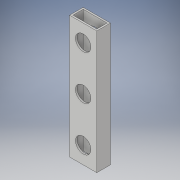
# Autodesk Inventor part: AluminumBar-1111-2020
Saved by Autodesk Inventor 2018 (Build 220112000, 112)
## iProperties
Created: 2020-01-25
Part Number: AluminumBar-1111-2020
Material: Generic
Document SubType Name: Modeling
Designer: Power Hawks CADD
Density: 1 g/cm^3
Appearance: Default
Author: Power Hawks CADD
Autodesk Inventor part; units mm, degrees
ref_plane "YZ Plane" through (0, 0, 0) normal (1, 0, 0) x (0, 1, 0)
ref_plane "XZ Plane" through (0, 0, 0) normal (0, 1, 0) x (-1, 0, 0)
ref_plane "XY Plane" through (0, 0, 0) normal (0, 0, 1) x (1, 0, 0)
sketch "Sketch2" plane through (0, 0, 0) normal (0, 1, 0) x (-1, 0, 0)
  line L0 (0, 0) -> (50.8, 0)
  line L1 (50.8, 0) -> (50.8, -25.4)
  line L2 (50.8, -25.4) -> (0, -25.4)
  line L3 (0, -25.4) -> (0, 0)
  line L4 (47.625, -22.225) -> (47.625, -3.175)
  line L5 (47.625, -3.175) -> (3.175, -3.175)
  line L6 (3.175, -3.175) -> (3.175, -22.225)
  line L7 (3.175, -22.225) -> (47.625, -22.225)
  dimension "d4" = 50.8
  dimension "d5" = 25.4
  dimension "d6" = 3.175
  constraints: 16 end point, 4 parallel, 2 perpendicular, 1 horizontal, 3 other
  measures "d4" distance of L1.end L2.end
  measures "d5" distance of L0.end L1.end
  measures "d6" distance between parallel lines of L1 L4
extrude "Extrusion2" add sketch "Sketch2" along normal blind 228.6
sketch "Sketch3" plane through (-50.8, 0, 0) normal (0, 0, 1) x (1, 0, 0)
  circle A0 centre (25.4, 31.75) radius 14.2875
  line L0 (50.8, 0) -> (0, 0) projected
  line L1 (0, 0) -> (0, 228.6) projected
  circle A1 centre (25.4, 196.85) radius 14.2875
  line L2 (0, 228.6) -> (50.8, 228.6) projected
  circle A2 centre (25.4, 114.3) radius 14.2875
  dimension "d9" = 31.75
  dimension "d10" = 25.4
  dimension "d11" = 25.4
  dimension "d12" = 31.75
  dimension "d13" = 114.3
  dimension "d14" = 25.4
  dimension "d15" = 28.575
  dimension "d16" = 28.575
  dimension "d17" = 28.575
  constraints: 3 centre point
  measures "d9" distance from line of L0 A0.centre
  measures "d10" distance from line of L1 A0.centre
  measures "d11" distance from line of L1 A1.centre
  measures "d12" distance from line of L2 A1.centre
  measures "d13" distance from line of L0 A2.centre
  measures "d14" distance from line of L1 A2.centre
  measures "d15" diameter of A2
  measures "d16" diameter of A0
  measures "d17" diameter of A1
extrude "Extrusion3" cut sketch "Sketch3" against normal blind 50.8
body "Solid2"
